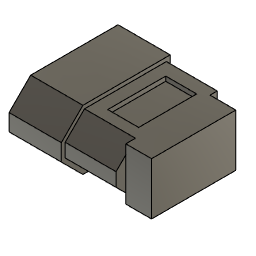
Comp_XT60F (Autodesk Fusion 360 design; units mm, degrees)
Autodesk Fusion 360 part; units mm, degrees
box "BoxPrimitive4" add length 15.7 width 8.2 height 8.1 placed x (0, 1, 0) y (-1, 0, 0) z (0, 0, 1) at (8.2, 0, 0) makes body 1 in component "XT60F"
chamfer "Chamfer4" distance 3 angle 45 2 edges at (4.1, 0, 0) (4.1, 0, 8.1) on bodies 1 in component "XT60F"
cylinder "CylinderPrimitive1" add diameter 6 height 4 placed x (0, 0, -1) y (0, 1, 0) z (1, 0, 0) at (8.2, 3, 4) separate body makes body 2 in component "XT60F"
move_body "Align3" bodies 2 to x (1, 0, 0) y (0, 1, 0) z (0, 0, 1) at (0, 4.85, 0.05) in component "XT60F"
move_body "Move6" bodies 2 to x (1, 0, 0) y (0, 1, 0) z (0, 0, 1) at (0, -3.35, 0) in component "XT60F"
copy_body "CopyPasteBodies4" bodies 2 makes body 3 in component "XT60F"
move_body "Move7" bodies 3 to x (1, 0, 0) y (0, 1, 0) z (0, 0, 1) at (0, 7, 0) in component "XT60F"
box "BoxPrimitive5" add length 9 width 4.8 height 0.7 placed x (0, -1, 0) y (1, 0, 0) z (0, 0, 1) at (3.4, 15.7, 8.1) separate body makes body 4 in component "XT60F"
box "BoxPrimitive6" add length 8.5 width 2.5 height -0.2 placed x (0, 1, 0) y (-1, 0, 0) z (0, 0, 1) at (6.9347, 6.5752, 8.8) separate body makes body 5 in component "XT60F"
move_body "Move8" bodies 4 5 to x (1, 0, 0) y (0, 1, 0) z (0, 0, 1) at (-1.2, -2, -0.7) in component "XT60F"
combine "Combine2" operation add target body 1 tool bodies 2 3 in component "XT60F"
copy_body "CopyPasteBodies6" bodies 5 4 makes body 6 makes body 7 in component "XT60F"
move_body "Move12" bodies 6 7 to x (1, 0, 0) y (0, 1, 0) z (0, 0, 1) at (0, 0, -11) in component "XT60F"
delete_body "RemoveBody1" bodies 5 in component "XT60F"
delete_body "RemoveBody2" bodies 6 in component "XT60F"
combine "Combine4" operation cut target body 1 tool bodies 4 in component "XT60F"
move_body "Move15" bodies 7 to x (1, 0, 0) y (0, 1, 0) z (0, 0, 1) at (0, 0, 3.6) in component "XT60F"
combine "Combine11" operation cut target body 1 tool bodies 7 in component "XT60F"
move_face "OffsetFaces1" offset 7.8 1 faces at (0, 11.4667, 2.7) on bodies 1 in component "XT60F"
ref_plane "WorkPlane1" through (0.3, 7.85, 4.05) normal (1, 0, 0) x (0, 0, -1)
split "Split1" by plane through (0.3, 7.85, 4.05) normal (1, 0, 0) bodies 1 makes body 8 at (9.5333, 4.2013, 1.0649) in component "XT60F"
move_face "OffsetFaces2" offset 0.3 6 faces at (-5.1, 7.2333, 8.1) (-5.1, 1, 6.1) (-5.1, 0, 4.4) (-5.1, 1, 2) (-5.1, 7.2333, 0) (-5.1, 15.7, 5.4) on bodies 1 in component "XT60F"
combine "Combine12" operation add target body 1 tool bodies 8 in component "XT60F"
box "BoxPrimitive7" add length 8.1 width 11.575 height 4 placed x (0, 0, -1) y (0, 1, 0) z (1, 0, 0) at (8.2, 3, 8.1) bodies 1 in component "XT60F"
move_face "OffsetFaces3" offset 0.3 6 faces at (-5.1, 7.2505, 8.4) (-5.1, 0.7586, 6.2828) (-2.4, -0.3, 3.6586) (-2.4, 16, 2.6) (-2.4, 11.6252, -0.3) (-2.4, 1.8172, 0.7586) on bodies 1 in component "XT60F"
box "BoxPrimitive8" add length 8.1 width 4 height 1.5 placed x (0, 0, -1) y (1, 0, 0) z (0, -1, 0) at (8.2, 3, 8.1) bodies 1 in component "XT60F"
component "XT60F" placed x (1, 0, 0) y (0, 1, 0) z (0, 0, 1) at (0, 0, 0)
